Autodesk Inventor part; units mm, degrees
(part 2 of 2)
sketch "Sketch25" plane through (-9, -9, 8.651) normal (-1, 0, 0) x (0, 0, 1)
  line L0 (-8.2995, 1.3) -> (-1.7005, 1.3) projected
  line L1 (-8.2995, 7.7) -> (-8.2995, 1.3) projected
  line L2 (-1.7005, 7.7) -> (-8.2995, 7.7) projected
  line L3 (-1.7005, 1.3) -> (-1.7005, 7.7) projected
  line L4 (-8.2995, -95.7) -> (-1.7005, -95.7) projected
  line L5 (-8.2995, -89.3) -> (-8.2995, -95.7) projected
  line L6 (-1.7005, -89.3) -> (-8.2995, -89.3) projected
  line L7 (-1.7005, -95.7) -> (-1.7005, -89.3) projected
  point P0 (-8.651, 9)
extrude "Extrusion28" cut sketch "Sketch25" against normal blind 9
sketch "Sketch26" plane through (0, 0, 1.651) normal (0, 0, 1) x (1, 0, 0)
  circle A0 centre (73.6502, -92.18) radius 3.05 projected
  line L0 (68.3002, -100.58) -> (68.3002, -83.78) projected
  line L1 (79.0002, -100.58) -> (68.3002, -100.58) projected
  line L2 (79.0002, -83.78) -> (79.0002, -100.58) projected
  line L3 (68.3002, -83.78) -> (79.0002, -83.78) projected
  line L4 (69.9002, -85.38) -> (69.9002, -98.98) projected
  line L5 (69.9002, -98.98) -> (77.4002, -98.98) projected
  line L6 (77.4002, -98.98) -> (77.4002, -85.38) projected
  line L7 (77.4002, -85.38) -> (69.9002, -85.38) projected
  point P0 (0, 0)
sketch "Sketch27" plane through (0, 0, 1.651) normal (0, 0, 1) x (1, 0, 0)
  circle A0 centre (104.8902, -84.37) radius 3.05
  line L0 (99.5402, -92.77) -> (99.5402, -75.97)
  line L1 (110.2402, -92.77) -> (99.5402, -92.77)
  line L2 (110.2402, -75.97) -> (110.2402, -92.77)
  line L3 (99.5402, -75.97) -> (110.2402, -75.97)
  line L4 (101.1402, -77.57) -> (101.1402, -91.17)
  line L5 (101.1402, -91.17) -> (108.6402, -91.17)
  line L6 (108.6402, -91.17) -> (108.6402, -77.57)
  line L7 (108.6402, -77.57) -> (101.1402, -77.57)
  circle A1 centre (104.8902, -84.37) radius 6.22 projected
  point P0 (0, 0)
  point P1 (0, 0)
  constraints: 16 end point, 1 centre point
extrude "Extrusion29" add sketch "Sketch27" against normal blind 1.651 contours A0 | A1 L0 | L0 A1 L4 | L4 A1 L6 | A1 L6 L2 | L2 A1
extrude "Extrusion30" add sketch "Sketch27" along normal up to surface (4.65 mm away) contours A0 | L0 A1 L4 L5 L6 L2 L1 | L0 A1 L4 | L0 L3 L2 A1 L6 L7 L4 | A1 L6 L5 L4 | L4 A1 L6 | A1 L6 L2 | L4 L7 L6 A1
extrude "Extrusion31" cut sketch "Sketch27" along normal up to surface (3 mm away) contours A0 | A1 L6 L5 L4 | L4 A1 L6 | L4 L7 L6 A1
extrude "Extrusion32" cut sketch "Sketch27" against normal blind 10 contours A0 | A1 L6 L5 L4 | L4 A1 L6 | L4 L7 L6 A1
extrude "Extrusion33" cut sketch "Sketch27" along normal blind 10 contours A0
body "Solid1"
